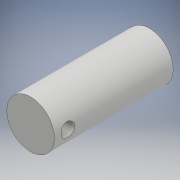
# Autodesk Inventor part: tige
Saved by Autodesk Inventor 2018 (Build 220112000, 112)
## iProperties
Created: 2018-02-07
Part Number: tige
Material: Générique
Document SubType Name: Modeling
Designer: Mephiro
Density: 1 g/cm^3
Appearance: Par défaut
Author: Mephiro
Autodesk Inventor part; units mm, degrees
ref_plane "YZ Plane" through (0, 0, 0) normal (1, 0, 0) x (0, 1, 0)
ref_plane "XZ Plane" through (0, 0, 0) normal (0, 1, 0) x (-1, 0, 0)
ref_plane "XY Plane" through (0, 0, 0) normal (0, 0, 1) x (1, 0, 0)
sketch "Esquisse1" plane through (0, 0, 0) normal (0, 1, 0) x (-1, 0, 0)
  circle A0 centre (0, 0) radius 7
  dimension "d0" = 14
  constraints: 1 centre point, 1 coincident
  measures "d0" diameter of A0
extrude "Extrusion1" add sketch "Esquisse1" along normal blind 35
sketch "Esquisse2" plane through (0, 0, 0) normal (1, 0, 0) x (0, 1, 0)
  circle A0 centre (4, 0) radius 2.05
  line L0 (0, 7) -> (0, -7) projected
  point P0 (0, 0)
  dimension "d3" = 4.1
  dimension "d6" = 4
  constraints: 1 centre point
  measures "d3" diameter of A0
  measures "d6" distance from line of L0 A0.centre
extrude "Extrusion2" cut sketch "Esquisse2" along normal mid plane 30
